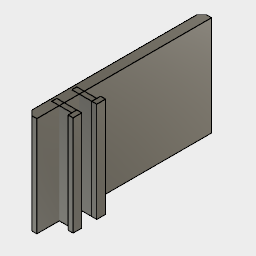
t-slot_cable_cover_v2_double_wide v0 (Autodesk Fusion 360 design; units mm, degrees)
Autodesk Fusion 360 part; units mm, degrees
box "BoxPrimitive1" add length 35 width 20 height 2 placed x (0, 1, 0) y (-1, 0, 0) z (0, 0, 1) at (20, 0, 0) makes body 1
box "BoxPrimitive4" add length 1 width 20 height 4 placed x (0, 1, 0) y (-1, 0, 0) z (0, 0, 1) at (20, 0, 0) separate body makes body 2
move_body "MoveBody4" bodies 2 to x (1, 0, 0) y (0, 1, 0) z (0, 0, 1) at (0, 5, 0)
copy_body "CopyPasteBodies2" bodies 2 makes body 3
move_body "MoveBody5" bodies 3 to x (1, 0, 0) y (0, 1, 0) z (0, 0, 1) at (0, 3, 0)
box "BoxPrimitive5" add length 1.75 width 20 height 1 placed x (0, 1, 0) y (-1, 0, 0) z (0, 0, 1) at (20, 0, 0) separate body makes body 4
move_body "MoveBody6" bodies 4 to x (1, 0, 0) y (0, 1, 0) z (0, 0, 1) at (0, 0, 5)
move_body "MoveBody7" bodies 4 to x (1, 0, 0) y (0, 1, 0) z (0, 0, 1) at (0, 4, 0)
move_body "MoveBody8" bodies 4 to x (1, 0, 0) y (0, 1, 0) z (0, 0, 1) at (0, 0, -1)
move_body "MoveBody9" bodies 4 to x (1, 0, 0) y (0, 1, 0) z (0, 0, 1) at (0, 0.5, 0)
copy_body "CopyPasteBodies3" bodies 4 makes body 5
move_body "MoveBody10" bodies 5 to x (1, 0, 0) y (0, 1, 0) z (0, 0, 1) at (0, 3.5, 0)
move_body "MoveBody11" bodies 5 4 3 1 2 to x (0, 0, -1) y (0, 1, 0) z (1, 0, 0) at (15.5, 0, 24.5)
chamfer "Chamfer1" distance 1 angle 45 1 edges at (15.5, 0, 14.5) on bodies 1
chamfer "Chamfer2" distance 1 angle 45 1 edges at (15.5, 35, 14.5) on bodies 1
move_body "MoveBody12" bodies 4 to x (1, 0, 0) y (0, 1, 0) z (0, 0, 1) at (0, -0.25, 0)
move_body "MoveBody13" bodies 2 4 to x (1, 0, 0) y (0, 1, 0) z (0, 0, 1) at (0, -0.75, 0)
move_body "MoveBody14" bodies 3 5 to x (1, 0, 0) y (0, 1, 0) z (0, 0, 1) at (0, 0.75, 0)
move_body "MoveBody15" bodies 2 3 4 5 to x (1, 0, 0) y (0, 1, 0) z (0, 0, 1) at (0.5, 0, 0)
move_body "MoveBody16" bodies 2 4 to x (1, 0, 0) y (0, 1, 0) z (0, 0, 1) at (0, 0.25, 0)
move_body "MoveBody17" bodies 3 5 to x (1, 0, 0) y (0, 1, 0) z (0, 0, 1) at (0, -0.25, 0)
